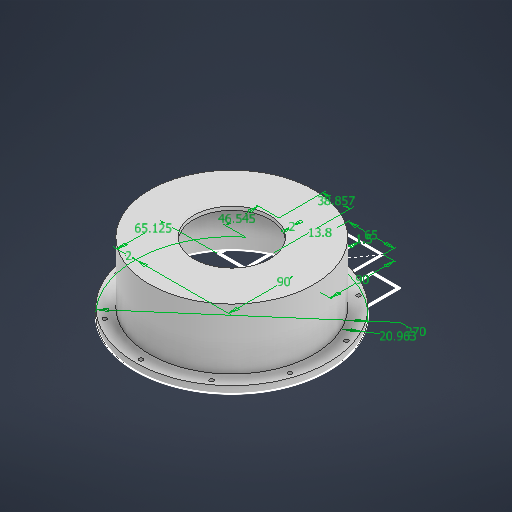
# Autodesk Inventor part: Cylinder  Segment - 01
Saved by Autodesk Inventor 2025 (Build 290162000, 162)
## iProperties
Created: 2024-04-11
Part Number: Cylinder  Segment - 01
Material: Generic
Document SubType Name: Modeling
Designer: Thienan Hoang
Density: 1 g/cm^3
Appearance: Default
Author: Thienan Hoang
Autodesk Inventor part; units mm, degrees
ref_plane "YZ Plane" through (0, 0, 0) normal (1, 0, 0) x (0, 1, 0)
ref_plane "XZ Plane" through (0, 0, 0) normal (0, 1, 0) x (-1, 0, 0)
ref_plane "XY Plane" through (0, 0, 0) normal (0, 0, 1) x (1, 0, 0)
sketch "Sketch1" plane through (0, 0, 0) normal (0, 1, 0) x (-1, 0, 0)
  circle A0 centre (0, 0) radius 135
  circle A1 centre (0, 0) radius 115
  circle A2 centre (0, 0) radius 112.0375
  circle A3 centre (0, 0) radius 9.5
  dimension "Absolute_Diameter" = 270
  dimension "Diameter_No_Outer_Lip" = 230
  dimension "Inner_Cylinder_Diameter" = 224.075
  dimension "Lip_Diameter" = 19
  constraints: 4 centre point, 4 coincident
  measures "Absolute_Diameter" diameter of A0
  measures "Diameter_No_Outer_Lip" diameter of A1
  measures "Inner_Cylinder_Diameter" diameter of A2
  measures "Lip_Diameter" diameter of A3
extrude "Extrusion1" add sketch "Sketch1" along normal blind 10 contours A0
extrude "Extrusion2" add sketch "Sketch1" along normal blind 95 contours A1
sketch "Sketch2" plane through (0, 95, 0) normal (0, 1, 0) x (1, 0, 0)
  circle A0 centre (0, 0) radius 115
  circle A1 centre (0, 0) radius 53.125
  dimension "Lip_Diameter_Out" = 230
  dimension "Inner_Lip_Diameter" = 106.25
  constraints: 2 centre point, 1 coincident
  measures "Lip_Diameter_Out" diameter of A0
  measures "Inner_Lip_Diameter" diameter of A1
extrude "Extrusion7" add sketch "Sketch2" against normal blind 5
ref_plane "Work Plane2" through (0, 10, 0) normal (0, 1, 0) x (1, 0, 0)
sketch "Sketch3" plane through (0, 10, 0) normal (0, 1, 0) x (1, 0, 0)
  circle A0 centre (0, 0) radius 127.5
  circle A1 centre (0, 127.5) radius 2.75
  circle A2 centre (-74.9426, 103.1497) radius 2.75
  circle A3 centre (-121.2597, 39.3997) radius 2.75
  circle A4 centre (-121.2597, -39.3997) radius 2.75
  circle A5 centre (-74.9426, -103.1497) radius 2.75
  circle A6 centre (0, -127.5) radius 2.75
  circle A7 centre (74.9426, -103.1497) radius 2.75
  circle A8 centre (121.2597, -39.3997) radius 2.75
  circle A9 centre (121.2597, 39.3997) radius 2.75
  circle A10 centre (74.9426, 103.1497) radius 2.75
  dimension "d27" = 255
  dimension "d229" = 5.5
  dimension "d232" = 360
  constraints: 10 centre point, 1 coincident, 1 vertical alignment, 23 other
  measures "d229" diameter of A1
extrude "Extrusion8" cut sketch "Sketch3" against normal blind 10 contours A9 A0 | A0 A9 | A8 A0 | A0 A8 | A10 A0 | A0 A10 | A7 A0 | A0 A7 | A1 A0 | A0 A1 | A6 A0 | A0 A6 | A2 A0 | A0 A2 | A5 A0 | A0 A5 | A3 A0 | A0 A3 | A4 A0 | A0 A4
sketch "Sketch24" plane through (0, 0, 0) normal (0, -1, 0) x (1, 0, 0)
  circle A0 centre (0, 0) radius 112.0375
  arc A1 (-85.157, -104.7535) -> (32.5, -131.0296) centre (0, 0) ccw
  circle A2 centre (0, 0) radius 133
  line L0 (-32.5, -90) -> (32.5, -90)
  line L1 (32.5, -90) -> (32.5, -180)
  line L2 (32.5, -180) -> (-32.5, -180)
  line L3 (-32.5, -180) -> (-32.5, -90)
  line L4 (-32.5, -90) -> (32.5, -180) construction
  line L5 (32.5, -90) -> (-32.5, -180) construction
  line L6 (-31, -178.5) -> (31, -178.5)
  line L7 (31, -178.5) -> (31, -91.5)
  line L8 (31, -91.5) -> (-31, -91.5)
  line L9 (-31, -91.5) -> (-31, -178.5)
  line L10 (-85.157, -65.125) -> (-46.3, -65.125)
  line L11 (-46.3, -65.125) -> (-46.3, -151.2985)
  line L12 (-46.3, -151.2985) -> (-85.157, -151.2985)
  line L13 (-85.157, -151.2985) -> (-85.157, -65.125)
  arc A3 (32.5, -131.0296) -> (-85.157, -104.7535) centre (0, 0) ccw
  line L14 (0, -91.5) -> (0, -178.5)
  line L15 (-83.157, -149.2985) -> (-48.3, -149.2985)
  line L16 (-48.3, -149.2985) -> (-48.3, -67.125)
  line L17 (-48.3, -67.125) -> (-83.157, -67.125)
  line L18 (-83.157, -67.125) -> (-83.157, -149.2985)
  line L19 (85.157, -65.125) -> (46.3, -65.125)
  line L20 (46.3, -65.125) -> (46.3, -151.2985)
  line L21 (46.3, -151.2985) -> (85.157, -151.2985)
  line L22 (85.157, -151.2985) -> (85.157, -65.125)
  line L23 (83.157, -149.2985) -> (48.3, -149.2985)
  line L24 (48.3, -149.2985) -> (48.3, -67.125)
  line L25 (48.3, -67.125) -> (83.157, -67.125)
  line L26 (83.157, -67.125) -> (83.157, -149.2985)
  point P0 (0, -135)
  dimension "d234" = 2
  dimension "d235" = 65
  dimension "d236" = 90
  dimension "d237" = 1.5
  dimension "d238" = 65.125
  dimension "d240" = 20.9625
  dimension "d241" = 270
  dimension "d242" = 90
  dimension "d243" = 13.8
  dimension "d244" = 38.857
  dimension "d246" = 46.545
  dimension "d247" = 2
  constraints: 54 end point, 8 parallel, 8 symmetric about line, 5 point on circle, 4 centre point, 4 midpoint, 4 perpendicular, 2 coincident, 2 horizontal, 2 point on line, 6 other
  measures "d234" radial gap between concentric circles of A1 A2
  measures "d235" distance of L1.end L2.end
  measures "d236" distance of L0.end L1.end
  measures "d237" distance between parallel lines of L2 L6
  measures "d238" distance from line of point (0, 0) L10
  measures "d240" radial gap between concentric circles of A2 A0
  measures "d241" diameter of A1
  measures "d242" distance from line of A0.centre L0
  measures "d243" distance between parallel lines of L3 L11
  measures "d244" distance of L11.end L12.end
  measures "d246" distance of A1.start L12.end
  measures "d247" distance between parallel lines of L12 L15
body "Solid1"
